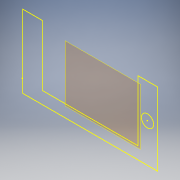
# Autodesk Inventor part: Bracket 2
Saved by Autodesk Inventor 2019 (Build 230136000, 136)
## iProperties
Created: 2020-07-29
Part Number: Bracket 2
Material: Generic
Document SubType Name: Modeling
Designer: Ian
Density: 1 g/cm^3
Appearance: Default
Author: Ian
Autodesk Inventor part; units mm, degrees
ref_plane "YZ Plane" through (0, 0, 0) normal (1, 0, 0) x (0, 1, 0)
ref_plane "Work Plane1" through (5, 0, 4.5) normal (0, 0, 1) x (1, 0, 0)
sketch "Sketch1" plane through (5, 0, 4.5) normal (0, 0, 1) x (1, 0, 0)
  circle A0 centre (25.5, 6.25) radius 1.5 projected
  line L0 (28, 14.65) -> (28, -27.65) projected
  line L1 (23.15, 14.65) -> (28, 14.65) projected
  line L2 (23.15, 14.65) -> (23.15, -0.15) projected
  line L3 (-0.15, -0.15) -> (23.15, -0.15) projected
  line L4 (-0.15, 14.65) -> (-0.15, -0.15) projected
  line L5 (-5, 14.65) -> (-0.15, 14.65) projected
  line L6 (-5, 14.65) -> (-5, -3.15) projected
  line L7 (23, -3.15) -> (-5, -3.15) projected
  circle A1 centre (25.5, -25.15) radius 1.5 projected
  circle A2 centre (-2.5, -25.15) radius 1.5 projected
  circle A3 centre (11.5, -25.15) radius 1.5 projected
  line L8 (23, -22.65) -> (23, -3.15) projected
  line L9 (23, -22.65) -> (-5, -22.65) projected
  line L10 (-5, -22.65) -> (-5, -27.65) projected
  line L11 (28, -27.65) -> (-5, -27.65) projected
  point P0 (-5, 0)
ref_plane "Work Plane2" through (28, 0, 0) normal (0, 0, 1) x (1, 0, 0)
extrude "Extrusion1" add sketch "Sketch1" against normal up to surface (4.5 mm away) contours L0 L11 L10 L9 L8 L7 L6 L5 L4 L3 L2 L1 | A1 | A2 | A3
sketch "Sketch2" plane through (33, -3.15, 0) normal (0, 0, -1) x (-1, 0, 0)
  circle A0 centre (2.5, 9.4) radius 1.5 projected
  line L0 (4.85, 17.8) -> (0, 17.8) projected
  line L1 (0, 17.8) -> (0, -24.5) projected
  line L2 (5, 0) -> (33, 0) projected
  line L3 (33, 0) -> (33, 17.8) projected
  line L4 (33, 17.8) -> (28.15, 17.8) projected
  line L5 (28.15, 17.8) -> (28.15, 3) projected
  line L6 (28.15, 3) -> (4.85, 3) projected
  line L7 (4.85, 3) -> (4.85, 17.8) projected
  line L8 (5, 15.65) -> (0, 15.65) projected
  line L9 (5, 3.15) -> (0, 3.15) projected
  line L10 (33, 15.65) -> (28, 15.65) projected
  line L11 (33, 3.15) -> (28, 3.15) projected
  line L12 (0, 17.8) -> (4.85, 17.8) projected
  line L13 (4.85, 17.8) -> (4.85, 3) projected
  line L14 (0, 17.8) -> (4.85, 17.8)
  line L15 (4.85, 17.8) -> (4.85, 15.65)
  line L16 (4.85, 15.65) -> (0, 15.65)
  line L17 (0, 15.65) -> (0, 17.8)
  line L18 (28.15, 17.8) -> (33, 17.8)
  line L19 (33, 17.8) -> (33, 15.65)
  line L20 (33, 15.65) -> (28.15, 15.65)
  line L21 (28.15, 15.65) -> (28.15, 17.8)
  line L22 (33, 0) -> (5, 0) projected
  line L23 (0, -24.5) -> (0, 17.8) projected
  line L24 (33, 0) -> (0, 0)
  line L25 (0, 0) -> (0, 3)
  line L26 (0, 3) -> (33, 3)
  line L27 (33, 3) -> (33, 0)
  line L28 (28.15, 3.15) -> (33, 3.15)
  line L29 (33, 3.15) -> (33, 3)
  line L30 (33, 3) -> (28.15, 3)
  line L31 (28.15, 3) -> (28.15, 3.15)
  line L32 (4.85, 3.15) -> (0, 3.15)
  line L33 (0, 3.15) -> (0, 3)
  line L34 (0, 3) -> (4.85, 3)
  line L35 (4.85, 3) -> (4.85, 3.15)
  line L36 (0, -24.5) -> (33, -24.5) projected
  line L37 (33, -24.5) -> (33, -19.5) projected
  line L38 (33, -19.5) -> (5, -19.5) projected
  line L39 (5, -19.5) -> (5, 0) projected
  constraints: 40 end point, 10 parallel, 7 point on line, 5 horizontal, 5 perpendicular
ref_plane "Work Plane3" through (0, -3.15, -2.5) normal (0, 0, 1) x (1, 0, 0)
extrude "Extrusion2" add sketch "Sketch2" along normal up to surface (2.5 mm away) contours L7 L8 L1 L0 | L7 L26 L1 L9 | L5 L11 L3 L26 | L5 L4 L3 L10
ref_plane "Work Plane5" through (11.25, 23, 12.45) normal (0, 0, 1) x (-1, 0, 0)
sketch "Sketch4" plane through (11.25, 23, 12.45) normal (0, 0, 1) x (-1, 0, 0)
  circle A0 centre (0, 0) radius 2.45 projected
  arc A1 (-21.75, -1) -> (-18.75, -4) centre (-18.75, -1) ccw projected
  line L0 (8.25, -4) -> (-18.75, -4) projected
  arc A2 (8.25, -4) -> (11.25, -1) centre (8.25, -1) ccw projected
  line L1 (11.25, 5.35) -> (11.25, -1) projected
  line L2 (6.4, 5.35) -> (11.25, 5.35) projected
  line L3 (6.4, 4) -> (6.4, 5.35) projected
  line L4 (-16.9, 4) -> (6.4, 4) projected
  line L5 (-16.9, 5.35) -> (-16.9, 4) projected
  line L6 (-21.75, 5.35) -> (-16.9, 5.35) projected
  line L7 (-21.75, -1) -> (-21.75, 5.35) projected
  point P0 (11.25, 23)
extrude "Extrusion3" add sketch "Sketch4" along normal blind 3
sketch "Sketch5" plane through (11.25, 23, 15.45) normal (0, 0, 1) x (1, 0, 0)
  line L0 (-6.4, -5.35) -> (-11.25, -5.35) projected
  line L1 (-6.4, -8.35) -> (-11.25, -8.35) projected
  line L2 (-11.25, -5.35) -> (-6.4, -5.35)
  line L3 (-6.4, -5.35) -> (-6.4, -8.35)
  line L4 (-6.4, -8.35) -> (-11.25, -8.35)
  line L5 (-11.25, -8.35) -> (-11.25, -5.35)
  line L6 (16.9, -5.35) -> (21.75, -5.35) projected
  line L7 (21.75, -8.35) -> (16.9, -8.35) projected
  line L8 (16.9, -5.35) -> (21.75, -5.35)
  line L9 (21.75, -5.35) -> (21.75, -8.35)
  line L10 (21.75, -8.35) -> (16.9, -8.35)
  line L11 (16.9, -8.35) -> (16.9, -5.35)
  circle A0 centre (19.25, -16.75) radius 1.5 projected
  line L12 (21.75, -50.65) -> (21.75, -8.35) projected
  line L13 (21.75, -8.35) -> (16.9, -8.35) projected
  line L14 (16.9, -8.35) -> (16.9, -23.15) projected
  line L15 (16.9, -23.15) -> (-6.4, -23.15) projected
  line L16 (-6.4, -23.15) -> (-6.4, -8.35) projected
  line L17 (-6.4, -8.35) -> (-11.25, -8.35) projected
  line L18 (-11.25, -8.35) -> (-11.25, -26.15) projected
  line L19 (-11.25, -26.15) -> (16.75, -26.15) projected
  line L20 (16.75, -26.15) -> (16.75, -45.65) projected
  line L21 (16.75, -45.65) -> (-11.25, -45.65) projected
  line L22 (-11.25, -45.65) -> (-11.25, -50.65) projected
  line L23 (-11.25, -50.65) -> (21.75, -50.65) projected
  point P0 (-11.25, -23)
  constraints: 16 end point, 4 parallel, 2 horizontal, 2 perpendicular
extrude "Extrusion4" add sketch "Sketch5" against normal blind 3
sketch "Sketch6" plane through (5, 0, 4.5) normal (0, 0, 1) x (1, 0, 0)
  line L0 (-5, 14.65) -> (-0.15, 14.65) projected
  circle A0 centre (25.5, 6.25) radius 1.5 projected
  line L1 (28, 14.65) -> (28, -27.65) projected
  line L2 (23.15, 14.65) -> (28, 14.65) projected
  line L3 (23.15, 14.65) -> (23.15, -0.15) projected
  line L4 (-0.15, -0.15) -> (23.15, -0.15) projected
  line L5 (-0.15, 14.65) -> (-0.15, -0.15) projected
  line L6 (-5, 14.65) -> (-0.15, 14.65) projected
  line L7 (-5, 14.65) -> (-5, -3.15) projected
  line L8 (23, -3.15) -> (-5, -3.15) projected
  circle A1 centre (6.25, 23) radius 10 projected
  circle A2 centre (6.25, 23) radius 12
  line L9 (-2.3684, 14.65) -> (-5, 14.65)
  line L10 (-5, 12.5) -> (-5, 14.65) projected
  line L11 (-5, 14.65) -> (-5, 12.5)
  line L12 (-0.15, 12.5) -> (-5, 12.5) projected
  line L13 (-5, 12.5) -> (-0.15, 12.5)
  line L14 (-0.15, 12.5) -> (-0.15, 12.8491)
  line L15 (-0.15, 14.65) -> (-0.15, 12.5) projected
  circle A3 centre (25.5, -25.15) radius 1.5 projected
  circle A4 centre (-2.5, -25.15) radius 1.5 projected
  circle A5 centre (11.5, -25.15) radius 1.5 projected
  line L16 (23, -22.65) -> (23, -3.15) projected
  line L17 (23, -22.65) -> (-5, -22.65) projected
  line L18 (-5, -22.65) -> (-5, -27.65) projected
  line L19 (28, -27.65) -> (-5, -27.65) projected
  point P0 (-5, 0)
  dimension "d8" = 2
  constraints: 8 end point, 3 collinear, 2 point on circle, 2 point on line, 1 centre point
  measures "d8" radial gap between concentric circles of A1 A2
extrude "Extrusion5" add sketch "Sketch6" along normal up to surface (7.95 mm away) contours L0 A2 L5 L12 L7 | L12 L5 L4 L3 L2 L1 L19 L18 L17 L16 L8 L7 | A3 | A4 | A5
sketch "Sketch7" plane through (33, 0, 0) normal (1, 0, 0) x (0, 0, -1)
  line L0 (-15.45, -3.15) -> (0, -3.15) projected
  line L1 (-15.45, -3.15) -> (2.5, -3.15)
  line L2 (2.5, -3.15) -> (2.5, -22.65)
  line L3 (2.5, -22.65) -> (-15.45, -22.65)
  line L4 (-15.45, -22.65) -> (-15.45, -3.15)
  line L5 (-15.45, 4.75) -> (0, 4.75) projected
  line L6 (-12.45, 24) -> (-12.45, 14.65) projected
  line L7 (-12.45, 24) -> (-15.45, 24) projected
  line L8 (-15.45, 24) -> (-15.45, -27.65) projected
  line L9 (2.5, 0) -> (2.5, -0.15) projected
  line L10 (0, 0) -> (2.5, 0) projected
  line L11 (0, 12.5) -> (0, 0) projected
  line L12 (0, 12.5) -> (2.5, 12.5) projected
  line L13 (2.5, 14.65) -> (2.5, 12.5) projected
  line L14 (-12.45, 14.65) -> (2.5, 14.65) projected
  line L15 (-15.45, -22.65) -> (2.5, -22.65)
  line L16 (2.5, -22.65) -> (2.5, -27.65)
  line L17 (2.5, -27.65) -> (-15.45, -27.65)
  line L18 (-15.45, -27.65) -> (-15.45, -22.65)
  line L19 (0, -0.15) -> (0, -27.65) projected
  line L20 (0, -0.15) -> (2.5, -0.15) projected
  line L21 (-15.45, -27.65) -> (0, -27.65) projected
  point P0 (0, 0)
  point P1 (2.5, -3.15)
  dimension "d11" = 19.5
  dimension "d13" = 5
  constraints: 16 end point, 4 parallel, 2 collinear, 2 horizontal, 2 perpendicular
  measures "d11" distance of L3.end L0.start
  measures "d13" distance between parallel lines of L3 L17
extrude "Extrusion6" add sketch "Sketch7" against normal blind 5 contours L0 L19 L3 L4 | L1 L2 L3 L19 | L3 L19 L17 L8 | L3 L16 L17 L19
extrude "Extrusion7" add sketch "Sketch7" against normal up to surface (33 mm away) contours L3 L19 L17 L8 | L3 L16 L17 L19
sketch "Sketch8" plane through (33, -27.65, -2.5) normal (0, 0, -1) x (-1, 0, 0)
  circle A0 centre (2.5, 2.5) radius 1.65
  circle A1 centre (16.5, 2.5) radius 1.65
  circle A2 centre (30.5, 2.5) radius 1.65
  line L0 (2.5, 2.5) -> (16.5, 2.5) construction
  line L1 (16.5, 2.5) -> (30.5, 2.5) construction
  line L2 (0, 0) -> (33, 0) construction
  line L3 (0, 0) -> (0, 24.5) construction
  line L4 (33, 0) -> (33, 5) construction
  point P0 (33, 27.65)
  dimension "d18" = 3.3
  dimension "d19" = 3.3
  dimension "d20" = 3.3
  dimension "d21" = 2.5
  dimension "d22" = 2.5
  dimension "d23" = 2.5
  constraints: 4 end point, 3 centre point, 2 horizontal, 1 collinear
  measures "d18" diameter of A0
  measures "d19" diameter of A1
  measures "d20" diameter of A2
  measures "d21" distance between parallel lines of L2 L0
  measures "d22" distance from line of L3 L0.start
  measures "d23" distance from line of L4 L1.end
extrude "Extrusion8" cut sketch "Sketch8" against normal blind 2.5
body "Solid1"
